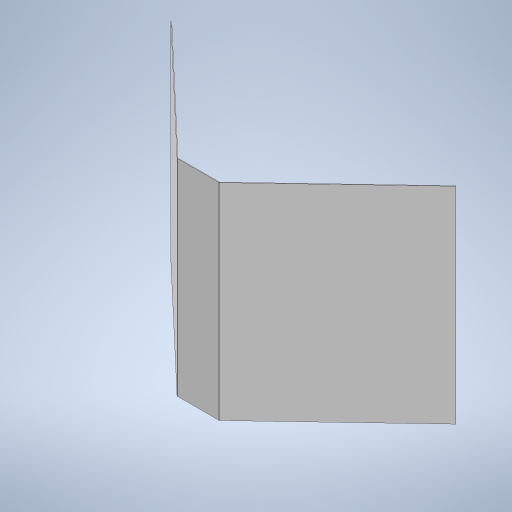
# Autodesk Inventor part: МОО 030 лист брюхо 1
Saved by Autodesk Inventor 2024.2 (Build 282272000, 272)
## iProperties
Created: 2024-04-28
Part Number: МОО 030 лист брюхо 1
Material: Stainless Steel
Document SubType Name: Sheet Metal
Designer: admin
Density: 8 g/cm^3
Flat Pattern Width: 100 cm
Flat Pattern Length: 182.761 cm
Flat Pattern Area: 18276.1 cm^2
Sheet Metal Rule: Default_mm
Sheet Metal Width: 1000,000 mm
Sheet Metal Length: 1827,612 mm
Sheet Metal Area: 1827612,056 mm^2
Appearance: Default
Mass: 43869.2 g
Surface Area: 36727.4 cm^2
Volume: 5483.66 cm^3
Author: admin
Autodesk Inventor part; units mm, degrees
ref_plane "YZ Plane" through (0, 0, 0) normal (1, 0, 0) x (0, 1, 0)
ref_plane "XZ Plane" through (0, 0, 0) normal (0, 1, 0) x (-1, 0, 0)
ref_plane "XY Plane" through (0, 0, 0) normal (0, 0, 1) x (1, 0, 0)
sketch "Sketch1" plane through (0, 0, 0) normal (0, 0, 1) x (1, 0, 0)
  line L0 (-100, 0) -> (100, 0)
  line L1 (0, 0) -> (0, 200) construction
  arc A0 (-102.0651, 0.8239) -> (-100, 0) centre (-100, 3) ccw
  line L2 (-102.0651, 0.8239) -> (-690, 558.7533)
  arc A1 (100, 0) -> (102.0651, 0.8239) centre (100, 3) ccw
  line L3 (102.0651, 0.8239) -> (690, 558.7533)
  dimension "d0" = 200
  dimension "d3" = 3
  dimension "d4" = 43.5
  dimension "d6" = 1380
  dimension "d18" = 810.5262
  measures "d0" distance of L0.start L0.end
  measures "d3" radius of A0
  measures "d4" angle of L0 L2
  measures "d6" distance of L3.end L2.end
  measures "d18" distance of L2.start L2.end
contour flange "Contour Flange1" sketch "Sketch1" thickness 3 bend radius 3 width 1000 along (0, 0, 1) mid plane no both sides no wall seen from (-396.0325, 279.7886, 0) lies toward (-0.6883546, -0.7253744, 0) curves L2 A0 L0 A1 L3
bend "Bend1"
corner "Corner1"
equation "\"d3\" = BendRadius"
equation "\"d7\" = Thickness"
equation "\"d8\" = BendReliefWidth"
equation "\"d9\" = BendReliefDepth"
equation "\"d10\" = MinimumRemnant"
equation "\"d11\" = TransitionRadius"
equation "\"d13\" = BendRadius"
equation "\"d15\" = CornerReliefSize"
equation "\"d16\" = GapSize"
equation "\"d17\" = JacobiRadiusSize"
equation "\"BendRadius\" = Thickness"
equation "\"BendReliefWidth\" = Thickness"
equation "\"BendReliefDepth\" = 0.5 * Thickness"
equation "\"CornerReliefSize\" = 4 * Thickness"
equation "\"MinimumRemnant\" = 2 * Thickness"
equation "\"TransitionRadius\" = BendRadius"
equation "\"JacobiRadiusSize\" = BendRadius"
equation "\"GapSize\" = Thickness"
equation "\"Thickness\" = 3"
body "Solid1"
